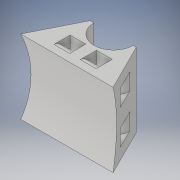
# Autodesk Inventor part: VHF_platform
Saved by Autodesk Inventor 2017 (Build 210142000, 142)
## iProperties
Created: 2018-06-16
Part Number: VHF_platform
Material: Generic
Document SubType Name: Modeling
Designer: Arthur
Density: 1 g/cm^3
Appearance: Default
Author: Arthur
Autodesk Inventor part; units mm, degrees
ref_plane "YZ Plane" through (0, 0, 0) normal (1, 0, 0) x (0, 1, 0)
ref_plane "XZ Plane" through (0, 0, 0) normal (0, 1, 0) x (-1, 0, 0)
ref_plane "XY Plane" through (0, 0, 0) normal (0, 0, 1) x (1, 0, 0)
sketch "Sketch1" plane through (0, 0, 0) normal (1, 0, 0) x (0, 1, 0)
  line L0 (16, 10) -> (-16, 10)
  line L1 (-16, 10) -> (-16, -10)
  line L2 (-16, -10) -> (16, -10)
  line L3 (16, -10) -> (16, 10)
  line L4 (16, 10) -> (-16, -10) construction
  line L5 (-16, 10) -> (16, -10) construction
  point P0 (0, 0)
  dimension "d0" = 32
  dimension "d1" = 20
  constraints: 12 end point, 2 midpoint, 2 parallel, 1 horizontal, 1 perpendicular
  measures "d0" distance of L2.end L1.end
  measures "d1" distance of L1.end L0.end
extrude "Extrusion1" add sketch "Sketch1" along normal blind 40
sketch "Sketch2" plane through (40, 0, 0) normal (1, 0, 0) x (0, 0, -1)
  line L0 (-10, 16) -> (-10, -16) projected
  line L1 (-10, 16) -> (-10, -16)
  arc A0 (-10, -16) -> (-10, 16) centre (-51.5241, 0) ccw
  point P0 (0, 0)
  dimension "d4" = 44.5
  constraints: 2 end point, 2 point on circle, 1 centre point, 1 collinear
  measures "d4" radius of A0
extrude "Extrusion2" cut sketch "Sketch2" against normal through all
sketch "Sketch3" plane through (0, 16, -10) normal (0, 1, 0) x (1, 0, 0)
  line L0 (11.6574, 0.0872) -> (28.6574, 0.0872)
  arc A0 (11.6574, 0.0872) -> (28.6574, 0.0872) centre (20.1574, 0.0872) ccw
  line L1 (0, -20) -> (0, 0) projected
  line L2 (10, 0) -> (0, -20)
  line L3 (0, -20) -> (0, 0)
  line L4 (0, 0) -> (10, 0)
  line L5 (40, 0) -> (40, -20) projected
  line L6 (30, 0) -> (40, -20)
  line L7 (40, -20) -> (40, 0)
  line L8 (30, 0) -> (40, 0)
  line L9 (0, 0) -> (40, 0) projected
  point P0 (0, -10)
  dimension "d8" = 17
  dimension "d36" = 10
  dimension "d37" = 10
  constraints: 14 end point, 2 point on circle, 1 centre point, 1 collinear, 1 horizontal, 1 perpendicular
  measures "d8" distance of L0.start L0.end
  measures "d36" distance of L1.end L2.start
  measures "d37" distance of L6.start L5.start
extrude "Extrusion3" cut sketch "Sketch3" against normal through all
sketch "Sketch6" plane through (20.1574, 16, -10.0872) normal (0, 1, 0) x (1, 0, 0)
  line L0 (8.4996, -0.0872) -> (9.8426, -0.0872) projected
  line L1 (-9.0815, -13.7992) -> (-2.2244, -13.7992)
  line L2 (-2.2244, -13.7992) -> (-2.2244, -9.7992)
  line L3 (-2.2244, -9.7992) -> (-9.0815, -9.7992)
  line L4 (-9.0815, -9.7992) -> (-9.0815, -13.7992)
  line L5 (9.2042, -13.7992) -> (2.3471, -13.7992)
  line L6 (2.3471, -13.7992) -> (2.3471, -9.7992)
  line L7 (2.3471, -9.7992) -> (9.2042, -9.7992)
  line L8 (9.2042, -9.7992) -> (9.2042, -13.7992)
  point P0 (-20.1574, -10.0872)
  point P1 (-8.4996, -0.0872)
  dimension "d39" = 4
  constraints: 16 end point, 4 parallel, 2 horizontal, 2 perpendicular
  measures "d39" distance of L3.end L1.start
extrude "Extrusion4" cut sketch "Sketch6" against normal through all
fillet "Fillet3" radius 3 4 edges at (14.5045, -16, 3.7121) (25.933, -16, 3.7121) (14.5045, 16, 3.7121) (25.933, 16, 3.7121)
sketch "Sketch7" plane through (10, -16, -10) normal (-0.8944272, 0, -0.4472136) x (-0.4472136, 0, 0.8944272)
  line L0 (15.3752, 4.9726) -> (10.8752, 4.9726)
  line L1 (10.8752, 4.9726) -> (10.8752, 11.9726)
  line L2 (10.8752, 11.9726) -> (15.3752, 11.9726)
  line L3 (15.3752, 11.9726) -> (15.3752, 4.9726)
  line L4 (15.3752, 26.9631) -> (10.8752, 26.9631)
  line L5 (10.8752, 26.9631) -> (10.8752, 19.9631)
  line L6 (10.8752, 19.9631) -> (15.3752, 19.9631)
  line L7 (15.3752, 19.9631) -> (15.3752, 26.9631)
  point P0 (13.4164, 16)
  dimension "d40" = 4.5
  dimension "d41" = 7
  dimension "d43" = 7
  constraints: 16 end point, 4 parallel, 2 horizontal, 2 perpendicular
  measures "d40" distance of L1.end L2.end
  measures "d41" distance of L0.end L1.end
  measures "d43" distance of L5.end L4.end
sketch "Sketch8" plane through (0, -16, 10) normal (0, -1, 0) x (1, 0, 0)
  line L0 (-11.5037, -8.1401) -> (42.8743, -8.1401)
  line L1 (0, 0) -> (40, 0) projected
  point P0 (0, -10)
  constraints: 2 end point, 1 horizontal, 1 parallel
sweep "Sweep2" cut profiles "Sketch7" path "Sketch8" path curves L0
fillet "Fillet4" radius 3 4 edges at (5.1365, -7.5274, -0.2729) (5.1365, 7.4631, -0.2729) (34.8635, -7.5274, -0.2729) (34.8635, 7.4631, -0.2729)
body "Solid1"
